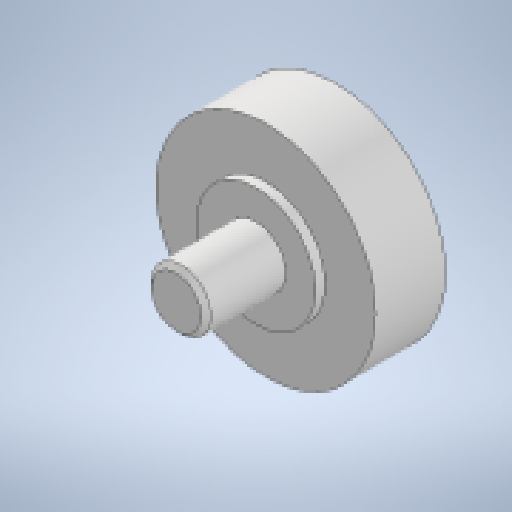
# Autodesk Inventor part: bearing 22-M6
Saved by Autodesk Inventor 2025 (Build 290162000, 162)
## iProperties
Created: 2025-04-20
Part Number: bearing 22-M6
Material: 一般
Document SubType Name: Modeling
Designer: gavin
Density: 1 g/cm^3
Appearance: 預設
Author: gavin
Autodesk Inventor part; units mm, degrees
ref_plane "YZ Plane" through (0, 0, 0) normal (1, 0, 0) x (0, 1, 0)
ref_plane "XZ Plane" through (0, 0, 0) normal (0, 1, 0) x (-1, 0, 0)
ref_plane "XY Plane" through (0, 0, 0) normal (0, 0, 1) x (1, 0, 0)
sketch "草圖1" plane through (0, 0, 0) normal (0, 0, 1) x (1, 0, 0)
  circle A0 centre (0, 0) radius 11
  dimension "d0" = 22
  constraints: 1 centre point, 1 coincident
  measures "d0" diameter of A0
extrude "擠出1" add sketch "草圖1" along normal blind 7
sketch "草圖2" plane through (0, 0, 7) normal (0, 0, 1) x (1, 0, 0)
  circle A0 centre (0, 0) radius 5.95
  dimension "d3" = 11.9
  constraints: 1 centre point, 1 coincident
  measures "d3" diameter of A0
extrude "擠出2" add sketch "草圖2" along normal blind 1
sketch "草圖3" plane through (0, 0, 8) normal (0, 0, 1) x (1, 0, 0)
  circle A0 centre (0, 0) radius 3
  dimension "d6" = 6
  constraints: 1 centre point, 1 coincident
  measures "d6" diameter of A0
extrude "擠出3" add sketch "草圖3" along normal blind 8
chamfer "倒角1" distance 0.5 angle 45 1 edges at (-3, 0, 16)
